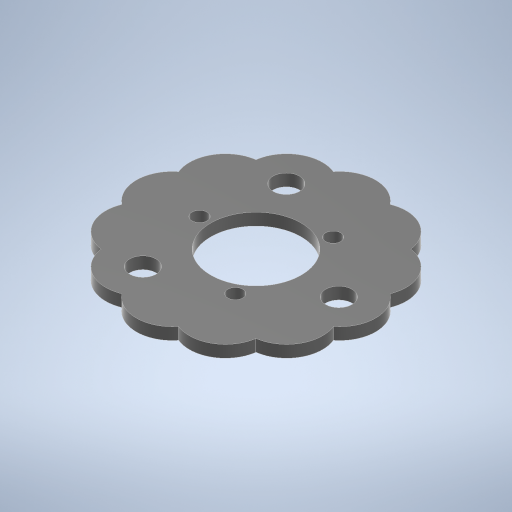
# Autodesk Inventor part: Motor Cap
Saved by Autodesk Inventor 2023.2 (Build 272271000, 271)
## iProperties
Created: 2022-12-29
Part Number: Motor Cap
Material: Nylon 6/6
Document SubType Name: Modeling
Designer: Nathan Cai
Density: 1.13 g/cm^3
Appearance: Smooth - Black
Mass: 1.4468 g
Surface Area: 19.2944 cm^2
Volume: 1.28035 cm^3
Author: Nathan Cai
Autodesk Inventor part; units mm, degrees
ref_plane "YZ Plane" through (0, 0, 0) normal (1, 0, 0) x (0, 1, 0)
ref_plane "XZ Plane" through (0, 0, 0) normal (0, 1, 0) x (-1, 0, 0)
ref_plane "XY Plane" through (0, 0, 0) normal (0, 0, 1) x (1, 0, 0)
sketch "Sketch1" plane through (0, 0, 0) normal (0, 1, 0) x (-1, 0, 0)
  circle A0 centre (0, 0) radius 6
  circle A1 centre (0, 0) radius 7.5 construction
  circle A2 centre (0, 0) radius 22.225 construction
  circle A3 centre (7.5, 0) radius 1
  line L0 (22.225, 0) -> (0, 0) construction
  circle A4 centre (-3.75, 6.4952) radius 1
  circle A5 centre (-3.75, -6.4952) radius 1
  circle A6 centre (0, 0) radius 17.4625
  dimension "d1" = 15
  dimension "d2" = 44.45
  dimension "d0" = 12
  dimension "d3" = 2
  dimension "d6" = 360
  dimension "d8" = 34.925
  constraints: 5 centre point, 4 coincident, 2 end point, 2 horizontal alignment, 1 horizontal, 1 point on line, 11 other
  measures "d0" diameter of A0
  measures "d3" diameter of A3
  measures "d8" diameter of A6
extrude "Extrusion1" add sketch "Sketch1" along normal blind 1.5875
sketch "Sketch2" plane through (0, 1.5875, 0) normal (0, 1, 0) x (1, 0, 0)
  circle A0 centre (0, 0) radius 11 construction
  line L0 (0, 0) -> (17.4625, 0) construction
  circle A1 centre (0, 0) radius 17.4625 projected
  circle A2 centre (11, 0) radius 1.7526
  circle A3 centre (-5.5, 9.5263) radius 1.7526
  circle A4 centre (-5.5, -9.5263) radius 1.7526
  dimension "d11" = 22
  dimension "d12" = 3.5052
  dimension "d15" = 360
  constraints: 3 centre point, 2 end point, 2 horizontal alignment, 1 coincident, 1 horizontal, 1 point on line, 10 other
  measures "d12" diameter of A2
extrude "Extrusion2" cut sketch "Sketch2" against normal through all contours A2 | A3 | A4
sketch "Sketch3" plane through (0, 1.5875, 0) normal (0, 1, 0) x (1, 0, 0)
  line L0 (0, 0) -> (11.1125, 0) construction
  circle A0 centre (0, 0) radius 11.1125 construction
  circle A1 centre (11.1125, 0) radius 4.7625
  circle A2 centre (9.6237, 5.5562) radius 4.7625
  circle A3 centre (5.5562, 9.6237) radius 4.7625
  circle A4 centre (0, 11.1125) radius 4.7625
  circle A5 centre (-5.5563, 9.6237) radius 4.7625
  circle A6 centre (-9.6237, 5.5563) radius 4.7625
  circle A7 centre (-11.1125, 0) radius 4.7625
  circle A8 centre (-9.6237, -5.5562) radius 4.7625
  circle A9 centre (-5.5563, -9.6237) radius 4.7625
  circle A10 centre (0, -11.1125) radius 4.7625
  circle A11 centre (5.5562, -9.6237) radius 4.7625
  circle A12 centre (9.6237, -5.5563) radius 4.7625
  circle A13 centre (0, 0) radius 17.4625
  point P0 (10.2741, -10.2741)
  point P1 (3.7606, -14.0347)
  point P2 (-3.7606, -14.0347)
  point P3 (-10.2741, -10.2741)
  point P4 (-14.0347, -3.7606)
  point P5 (-14.0347, 3.7606)
  point P6 (-10.2741, 10.2741)
  point P7 (-3.7606, 14.0347)
  point P8 (3.7606, 14.0347)
  point P9 (10.2741, 10.2741)
  point P10 (14.0347, 3.7606)
  point P11 (14.0347, -3.7606)
  dimension "d19" = 22.225
  dimension "d20" = 9.525
  dimension "d23" = 360
  dimension "d25" = 34.925
  constraints: 13 centre point, 3 coincident, 2 end point, 1 horizontal, 1 horizontal alignment, 27 other
  measures "d20" diameter of A1
  measures "d25" diameter of A13
extrude "Extrusion3" cut sketch "Sketch3" against normal blind 25.4
body "Solid1"
